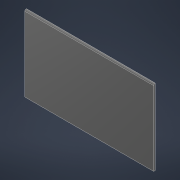
# Autodesk Inventor part: McCrea_plocha_walle
Saved by Autodesk Inventor 2022 (Build 260153000, 153)
## iProperties
Created: 2022-01-17
Part Number: McCrea_plocha_walle
Material: Rubber
Document SubType Name: Modeling
Designer: student
Density: 0.93 g/cm^3
Appearance: Dirt - Dark Brown
Author: student
Autodesk Inventor part; units mm, degrees
ref_plane "YZ Plane" through (0, 0, 0) normal (1, 0, 0) x (0, 1, 0)
ref_plane "XZ Plane" through (0, 0, 0) normal (0, 1, 0) x (-1, 0, 0)
ref_plane "XY Plane" through (0, 0, 0) normal (0, 0, 1) x (1, 0, 0)
sketch "Sketch1" plane through (0, 0, 0) normal (0, 0, 1) x (1, 0, 0)
  line L0 (-1432.7935, 866.3968) -> (267.2065, 866.3968)
  line L1 (267.2065, 866.3968) -> (267.2065, -133.6032)
  line L2 (267.2065, -133.6032) -> (-1432.7935, -133.6032)
  line L3 (-1432.7935, -133.6032) -> (-1432.7935, 866.3968)
  point P0 (0, 0)
  dimension "d0" = 1700
  dimension "d1" = 1000
  constraints: 8 end point, 2 parallel, 1 horizontal, 1 perpendicular
  measures "d0" distance of L1.end L2.end
  measures "d1" distance of L0.end L1.end
extrude "Extrusion1" add sketch "Sketch1" along normal blind 20
fillet "Fillet1" radius 20 1 edges at (-582.7935, 866.3968, 20)
body "Solid1"
